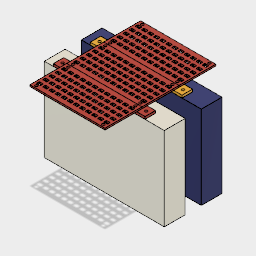
Master v11 (Autodesk Fusion 360 design; units mm, degrees)
Autodesk Fusion 360 part; units mm, degrees
note: some values were not read from the file. Set by a fixed rule: which face or edge a step refers to.
sketch "Sketch1" plane through (0, 0, 0) normal (0, 1, 0) x (1, 0, 0)
  line L0 (0.0413, -101.6, 101.6394) -> (0.0424, -101.6, 95.2894)
  line L1 (-28.4576, 6.3443) -> (-130.0576, 6.3473)
  line L2 (0.0413, -101.6, 101.6394) -> (0.0413, -101.6, 88.9394)
  line L3 (-23.4267, 12.6973) -> (-135.051, 12.6973)
  line L4 (-135.051, 12.6973) -> (-135.051, -0.0027)
  line L5 (-135.051, -0.0027) -> (-23.4267, -0.0027)
  line L6 (-23.4267, -0.0027) -> (-23.4267, 12.6973)
  line L7 (-28.4576, 6.3443) -> (-23.4576, 6.3447)
  line L8 (-130.0576, 6.3473) -> (-135.051, 6.3473)
  line L9 (-130.0576, 6.3473) -> (-135.0576, 6.3473)
  circle A0 centre (-130.0576, 6.3473) radius 1.5
  circle A1 centre (-28.4576, 6.3443) radius 1.5
  line L10 (-23.4267, 12.6973) -> (-38.4267, 12.6973)
  line L11 (-130.0576, 26.3473) -> (-135.051, 26.3473)
  circle A2 centre (-28.4576, 26.3443) radius 1.5
  line L12 (-28.4576, 26.3443) -> (-23.4576, 26.3447)
  circle A3 centre (-130.0576, 26.3473) radius 1.5
  line L13 (-135.051, 32.6973) -> (-135.051, 19.9973)
  line L14 (-23.4267, 19.9973) -> (-23.4267, 32.6973)
  line L15 (-23.4267, 32.6973) -> (-38.4267, 32.6973)
  line L16 (-130.0576, 26.3473) -> (-135.0576, 26.3473)
  line L17 (-28.4576, 26.3443) -> (-130.0576, 26.3473)
  line L18 (-23.4267, 32.6973) -> (-135.051, 32.6973)
  line L19 (-135.051, 19.9973) -> (-23.4267, 19.9973)
  dimension "d5" = 101.6
  dimension "d7" = 5
  dimension "d8" = 5
  dimension "d9" = 3
  dimension "d10" = 3
  dimension "d20" = 101.6
  dimension "d21" = 5
  dimension "d22" = 5
  dimension "d23" = 3
  dimension "d24" = 3
  measures "d5" distance of L1.start L1.end
  measures "d7" distance of L1.start L7.end
  measures "d8" distance of L1.end L9.end
  measures "d9" diameter of A0
  measures "d10" diameter of A1
  measures "d20" distance of L11.start A2.centre
  measures "d21" distance of A2.centre L12.end
  measures "d22" distance of L11.start L16.end
  measures "d23" diameter of A3
  measures "d24" diameter of A2
extrude "Extrude1" add sketch "Sketch1" along normal blind 3 contours L3 L4 L5 L6 L10 makes body 1
sketch "Sketch2" plane through (0, 0, 0) normal (0, 1, 0) x (1, 0, 0)
  line L0 (0, 0) -> (146, 0)
  line L1 (146, 0) -> (146, -25.4)
  line L2 (146, -25.4) -> (0, -25.4)
  line L3 (0, -25.4) -> (0, 0)
  line L4 (146, -25.4) -> (146, -19.05)
  line L5 (146, -19.05) -> (117.5, -19.05)
  line L6 (117.5, -19.05) -> (15.9, -19.05)
  circle A0 centre (15.9, -19.05) radius 1.4
  circle A1 centre (117.5, -19.05) radius 1.4
  circle A2 centre (117.5, -64.05) radius 1.4
  line L7 (0, -70.4) -> (0, -45)
  circle A3 centre (15.9, -64.05) radius 1.4
  line L8 (146, -64.05) -> (117.5, -64.05)
  line L9 (146, -70.4) -> (146, -64.05)
  line L10 (146, -70.4) -> (0, -70.4)
  line L11 (0, -45) -> (146, -45)
  line L12 (146, -45) -> (146, -70.4)
  line L13 (117.5, -64.05) -> (15.9, -64.05)
  point P0 (0, -45)
  dimension "d16" = 25.4
  dimension "d17" = 146
  dimension "d27" = 6.35
  dimension "d28" = 28.5
  dimension "d29" = 101.6
  dimension "d30" = 2.8
  dimension "d31" = 2.8
  dimension "d34" = 25.4
  dimension "d35" = 146
  dimension "d36" = 6.35
  dimension "d37" = 28.5
  dimension "d38" = 101.6
  dimension "d39" = 2.8
  dimension "d40" = 2.8
  measures "d16" distance of L0.start L2.end
  measures "d17" distance of L0.start L0.end
  measures "d27" distance of L1.end L4.end
  measures "d28" distance of L4.end L5.end
  measures "d29" distance of L5.end L6.end
  measures "d30" diameter of A0
  measures "d31" diameter of A1
  measures "d34" distance of P0 L7.start
  measures "d35" distance of P0 L11.end
  measures "d36" distance of L8.start L9.start
  measures "d37" distance of L8.start A2.centre
  measures "d38" distance of A3.centre A2.centre
  measures "d39" diameter of A3
  measures "d40" diameter of A2
extrude "Extrude4" add sketch "Sketch1" along normal blind 3 separate body contours L13 L14 L15 L18 L19 makes body 2
extrude "Extrude5" add sketch "Sketch2" along normal blind 101.6 separate body contours L0 L1 L2 L3 L4 makes body 3
move_body "Move1" bodies 1 to x (1, 0, 0) y (0, 1, 0) z (0, 0, 1) at (145, 100, 20)
move_body "Move2" bodies 1 to x (1, 0, 0) y (0, 1, 0) z (0, 0, 1) at (1, 0, 5.4)
extrude "Extrude6" add sketch "Sketch2" along normal blind 101.6 separate body contours L7 L9 L10 L11 L12 makes body 4
move_body "Move3" bodies 2 to x (1, 0, 0) y (0, 1, 0) z (0, 0, 1) at (126, 91, 65)
move_body "Move4" bodies 2 to x (1, 0, 0) y (0, 1, 0) z (0, 0, 1) at (0, 12, 0)
move_body "Move5" bodies 2 to x (1, 0, 0) y (0, 1, 0) z (0, 0, 1) at (0, -1.4, 16)
move_body "Move6" bodies 2 to x (1, 0, 0) y (0, 1, 0) z (0, 0, 1) at (20, 0, 9.3)
move_body "Move7" bodies 2 to x (1, 0, 0) y (0, 1, 0) z (0, 0, 1) at (0, 0, 0.1)
sketch "Sketch3" plane through (0, 0, 0) normal (0, 1, 0) x (1, 0, 0)
  line L0 (117.5, -64.05) -> (15.9, -64.05)
  line L1 (15.9, -19.05) -> (15.9, -64.05)
  line L2 (15.9, -19.05) -> (15.9, -22.05)
  line L3 (117.5, -19.05) -> (117.5, -22.05)
  line L4 (15.9, -64.05) -> (15.9, -61.05)
  line L5 (117.5, -64.05) -> (117.5, -61.05)
  line L6 (15.9, -22.05) -> (117.5, -22.05)
  line L7 (117.5, -22.05) -> (117.5, -61.05)
  line L8 (117.5, -61.05) -> (15.9, -61.05)
  line L9 (15.9, -61.05) -> (15.9, -22.05)
  line L10 (117.5, -22.05) -> (112.5, -22.05)
  line L11 (112.5, -22.05) -> (107.5, -22.05)
  line L12 (15.9, -22.05) -> (25.9, -22.05)
  circle A0 centre (25.9, -22.05) radius 1.5
  circle A1 centre (107.5, -22.05) radius 1.5
  line L13 (15.9, -61.05) -> (25.9, -61.05)
  line L14 (117.5, -61.05) -> (107.5, -61.05)
  circle A2 centre (25.9, -61.05) radius 1.5
  circle A3 centre (107.5, -61.05) radius 1.5
  line L15 (23.5, -55) -> (27.5, -55)
  line L16 (27.5, -55) -> (27.5, -57.5)
  line L17 (27.5, -57.5) -> (23.5, -57.5)
  line L18 (23.5, -57.5) -> (23.5, -55)
  point P0 (15.9, -19.05)
  point P1 (15.9, -64.05)
  point P2 (117.5, -19.05)
  dimension "d43" = 3
  dimension "d44" = 3
  dimension "d45" = 3
  dimension "d46" = 3
  dimension "d51" = 5
  dimension "d52" = 5
  dimension "d53" = 10
  dimension "d54" = 3
  dimension "d55" = 3
  dimension "d56" = 10
  dimension "d57" = 10
  dimension "d58" = 3
  dimension "d59" = 3
  dimension "d105" = 4
  dimension "d106" = 2.5
  measures "d43" distance of P0 L2.end
  measures "d44" distance of P2 L3.end
  measures "d45" distance of P1 L4.end
  measures "d46" distance of L0.start L5.end
  measures "d51" distance of L3.end L10.end
  measures "d52" distance of L10.end L11.end
  measures "d53" distance of L2.end L12.end
  measures "d54" diameter of A0
  measures "d55" diameter of A1
  measures "d56" distance of L4.end L13.end
  measures "d57" distance of L5.end L14.end
  measures "d58" diameter of A2
  measures "d59" diameter of A3
  measures "d105" distance of L15.start L15.end
  measures "d106" distance of L15.start L17.end
extrude "Extrude7" cut sketch "Sketch3" along normal blind 3 contours L1 L6 L7 L8 L9 L10 L11 L12 A0 A1 L13 L14 A2 A3 | L8 L14 A3 | L8 L13 A2 | L6 L12 A0 | L6 L11 A1 | L15 L16 L17 L18 picked at (106.7204, -60.4283) picked at (25.0364, -60.5514) picked at (26.8944, -22.1245) picked at (106.5056, -22.1245) bodies 3 4
extrude "Extrude8" add sketch "Sketch3" along normal blind 3 separate body contours L1 L6 L7 L8 L9 L10 L11 L12 A0 A1 L13 L14 A2 A3 | L8 L14 A3 | L8 L13 A2 | L6 L12 A0 | L6 L11 A1 | L15 L16 L17 L18 picked at (106.7204, -60.4283) picked at (25.0364, -60.5514) picked at (26.8944, -22.1245) picked at (106.5056, -22.1245) makes body 5
move_body "Move8" bodies 5 to x (1, 0, 0) y (0, 1, 0) z (0, 0, 1) at (0, 104.5, 0)
move_body "Move9" bodies 5 to x (1, 0, 0) y (0, 1, 0) z (0, 0, 1) at (0, 0.1, 0)
move_face "MoveFace1" by (-5, 0, 0) 1 faces at (117.5, 105.6, 35.05) on bodies 5
move_face "MoveFace2" by (5, 0, 0) 1 faces at (15.9, 105.6, 35.05) on bodies 5
move_face "MoveFace3" by (0, 0, 3) 7 faces at (111.3333, 105.6, 61.05) (108.5, 105.6, 61.05) (107, 105.6, 61.05) (79.8, 105.6, 61.05) (26.9, 105.6, 61.05) (25.4, 105.6, 61.05) (23.2333, 105.6, 61.05) on bodies 5
move_face "MoveFace4" by (0, 0, -3) 7 faces at (22.0667, 105.6, 22.05) (24.9, 105.6, 22.05) (26.4, 105.6, 22.05) (53.6, 106.6, 22.05) (106.5, 105.6, 22.05) (108, 105.6, 22.05) (110.1667, 105.6, 22.05) on bodies 5
move_body "Move10" bodies 1 to x (1, 0, 0) y (0, 1, 0) z (0, 0, 1) at (0, 2, 0)
move_body "Move11" bodies 1 to x (1, 0, 0) y (0, 1, 0) z (0, 0, 1) at (0, -0.4, 0)
move_face "MoveFace5" by (0, -1, 0) 1 faces at (79.8, 107.6, 49.05) on bodies 5
hole "Hole1" at (25.8896, 106.6, 21.9958) direction (0, -1, 0) diameter 3 depth 27 tip angle 118 bodies 1 3 5
hole "Hole2" at (107.5126, 106.6, 22.048) direction (0, -1, 0) diameter 3 depth 2 tip angle 118 bodies 1 5
hole "Hole3" at (107.5126, 104.6, 22.048) direction (0, -1, 0) diameter 3 depth 2 tip angle 118 bodies 1
hole "Hole4" at (25.9051, 106.6, 61.0462) direction (0, -1, 0) diameter 3 depth 2 tip angle 118 bodies 2 5
hole "Hole5" at (107.5057, 106.6, 61.0435) direction (0, -1, 0) diameter 3 depth 2 tip angle 118 bodies 2 5
hole "Hole6" at (25.9051, 104.6, 61.0462) direction (0, -1, 0) diameter 3 depth 2 tip angle 118 bodies 2
hole "Hole7" at (107.5057, 104.6, 61.0435) direction (0, -1, 0) diameter 3 depth 2 tip angle 118 bodies 2
copy_body "CopyPasteBodies1" bodies 5 makes body 6
move_body "Move12" bodies 6 to x (1, 0, 0) y (0, 1, 0) z (0, 0, 1) at (0, 0, 45)
hole "Hole8" at (25.8896, 106.6, 66.9958) direction (0, -1, 0) diameter 3 depth 2 tip angle 118 bodies 2
hole "Hole9" at (107.5126, 106.6, 67.048) direction (0, -1, 0) diameter 3 depth 2 tip angle 118 bodies 2
hole "Hole10" at (25.8896, 104.6, 66.9958) direction (0, -1, 0) diameter 3 depth 2 tip angle 118 bodies 2
hole "Hole11" at (107.5126, 104.6, 67.048) direction (0, -1, 0) diameter 3 depth 2 tip angle 118 bodies 2
hole "Hole12" at (25.8896, 104.6, 66.9958) direction (0, -1, 0) diameter 3 depth 3 tip angle 118 bodies 2 4
hole "Hole13" at (25.9051, 104.6, 61.0462) direction (0, -1, 0) diameter 3 depth 3 tip angle 118 bodies 2 4
hole "Hole14" at (107.5057, 104.6, 61.0435) direction (0, -1, 0) diameter 3 depth 3 tip angle 118 bodies 2 4
hole "Hole15" at (107.5126, 104.6, 67.048) direction (0, -1, 0) diameter 3 depth 3 tip angle 118 bodies 2 4
sketch "Sketch5" plane through (0, 106.6, 0) normal (0, 1, 0) x (-1, 0, 0)
  circle A0 centre (-107.5057, 61.0435) radius 1.5
  circle A1 centre (-25.9051, 61.0462) radius 1.5
  circle A2 centre (-107.5126, 22.048) radius 1.5
  circle A3 centre (-25.8896, 21.9958) radius 1.5
  line L0 (-20.9, 64.05) -> (-112.5, 64.05)
  line L1 (-112.5, 64.05) -> (-112.5, 19.05)
  line L2 (-112.5, 19.05) -> (-20.9, 19.05)
  line L3 (-20.9, 19.05) -> (-20.9, 64.05)
  line L4 (-23.5, 58.3) -> (-23.5, 55)
  line L5 (-15.9, 61.05) -> (-117.5, 61.05)
  line L6 (-23.5, 58.3) -> (-23.5, 61.05)
  line L7 (-23.5, 61.05) -> (-24.4051, 61.05)
  line L8 (-27.4051, 61.05) -> (-28.3101, 61.05)
  line L9 (-28.3101, 58.3) -> (-28.3101, 55)
  line L10 (-28.3101, 58.3) -> (-23.5, 58.3)
  line L11 (-28.3101, 55) -> (-23.5, 55)
  point P0 (-23.5, 55)
  dimension "d109" = 0.905
  measures "d109" distance of L8.start L8.end
extrude "Extrude9" cut sketch "Sketch5" against normal up to surface (5 mm away) contours L4 L9 L10 L11 bodies 5
fillet "Fillet1" radius 0.4 4 edges at (23.5, 105.6, 55) (23.5, 105.6, 58.3) (28.3101, 105.6, 58.3) (28.3101, 105.6, 55) on bodies 5
pattern_linear "R-Pattern1" count 12 spacing 7.4091 along (1, 0, 0) count 5 spacing 7.5 along (0, 0, -1) of "Extrude9", "Fillet1"
hole "Hole18" at (107.5, 0, 22.05) direction (0, 1, 0) diameter 3 depth 110 tip angle 118 bodies 1
copy_body "CopyPasteBodies2" bodies 6 makes body 7
move_body "Move13" bodies 7 to x (1, 0, 0) y (0, 1, 0) z (0, 0, 1) at (0, 0, -90)
hole "Hole20" at (107.5084, 104.6, 16.0472) direction (0, -1, 0) diameter 3 depth 2 tip angle 118 bodies 1
hole "Hole21" at (107.5084, 104.6, 16.0472) direction (0, -1, 0) diameter 3 depth 50 tip angle 118 bodies 1
hole "Hole22" at (25.9051, 106.6, 16.0462) direction (0, -1, 0) diameter 3 depth 50 tip angle 118 bodies 1
hole "Hole23" at (15.9424, 104.6, 19.0527) direction (0, -1, 0) diameter 3.2 depth 105 tip angle 118 bodies 1
hole "Hole24" at (117.5424, 104.6, 19.0557) direction (0, -1, 0) diameter 3.2 depth 11 tip angle 118 bodies 1
hole "Hole25" at (15.9424, 104.6, 64.0527) direction (0, -1, 0) diameter 3.2 depth 2 tip angle 118 bodies 2
hole "Hole26" at (117.5424, 104.6, 64.0557) direction (0, -1, 0) diameter 3.2 depth 2 tip angle 118 bodies 2
hole "Hole27" at (25.8896, 106.6, 21.9958) direction (0, -1, 0) diameter 3.2 depth 9 tip angle 118 bodies 1 5
hole "Hole28" at (25.9051, 104.6, 16.0462) direction (0, -1, 0) diameter 3.2 depth 11 tip angle 118 bodies 1
hole "Hole29" at (107.5126, 106.6, 22.048) direction (0, -1, 0) diameter 3.2 depth 11 tip angle 118 bodies 1 5
hole "Hole30" at (107.5084, 104.6, 16.0472) direction (0, -1, 0) diameter 3.2 depth 10 tip angle 118 bodies 1
hole "Hole31" at (25.9051, 106.6, 61.0462) direction (0, -1, 0) diameter 3.2 depth 8 tip angle 118 bodies 2 5
hole "Hole32" at (107.5057, 106.6, 61.0435) direction (0, -1, 0) diameter 3.2 depth 11 tip angle 118 bodies 2 5
hole "Hole33" at (25.8896, 104.6, 66.9958) direction (0, -1, 0) diameter 3.2 depth 12 tip angle 118 bodies 2
hole "Hole34" at (107.5126, 104.6, 67.048) direction (0, -1, 0) diameter 3.2 depth 9 tip angle 118 bodies 2
copy_body "CopyPasteBodies5" bodies 5 makes body 8
move_body "Move16" bodies 8 to x (1, 0, 0) y (0, 1, 0) z (0, 0, 1) at (0, 0, 45)
copy_body "CopyPasteBodies6" bodies 5 makes body 9
move_body "Move17" bodies 9 to x (1, 0, 0) y (0, 1, 0) z (0, 0, 1) at (0, 0, -45)
hidden bodies 6 7
